Autodesk Fusion 360 part; units mm, degrees
note: some values were not read from the file. Chosen so that the rebuilt part matches the saved one: which face or edge a step refers to; which pieces of a blend or face edit are solid. Set by a fixed rule: which sketch regions a step uses.
(part 2 of 2)
equation "d189 = lever"
equation "d191 = ( d188 - d190 ) / 2"
equation "d196 = hinge_bearing_innerdia"
equation "d197 = hinge_bearing_outerdia + 6 mm"
equation "d198 = d197 / 2"
equation "d199 = d198"
equation "d202 = d203"
equation "d204 = d203"
equation "d206 = d205"
equation "d238 = ( d237 - d236 ) / 2"
equation "d241 = d234 - 4 mm"
equation "d453 = d25"
equation "d462 = d461"
equation "d517 = d518"
equation "d518 = d682"
equation "d519 = d684 + 0.1 mm"
equation "d520 = d519"
equation "d543 = d542"
equation "d617 = d618 / 2"
equation "d620 = d619 / 2"
equation "d621 = d620"
equation "d623 = d622"
equation "d624 = d622"
equation "d625 = d622"
equation "d639 = d73"
equation "d640 = d639"
equation "d641 = d639"
equation "d642 = d119"
equation "d644 = d643"
equation "d646 = d117"
equation "d664 = d663"
equation "d671 = d670 + 0.2 mm"
equation "d690 = d689 + 2 mm"
